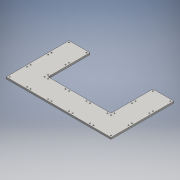
# Autodesk Inventor part: InnerFrame
Saved by Autodesk Inventor 2016 (Build 200138000, 138)
## iProperties
Created: 2016-05-22
Part Number: InnerFrame
Material: Generic
Document SubType Name: Modeling
Designer: Kurtis
Density: 1 g/cm^3
Appearance: Default
Author: Kurtis
Autodesk Inventor part; units mm, degrees
ref_plane "YZ Plane" through (0, 0, 0) normal (1, 0, 0) x (0, 1, 0)
ref_plane "XZ Plane" through (0, 0, 0) normal (0, 1, 0) x (-1, 0, 0)
ref_plane "XY Plane" through (0, 0, 0) normal (0, 0, 1) x (1, 0, 0)
sketch "Sketch1" plane through (0, 0, 0) normal (0, 0, 1) x (1, 0, 0)
  line L0 (0, 0) -> (0, 180)
  line L1 (0, 180) -> (60, 180)
  line L2 (60, 180) -> (60, 60)
  line L3 (60, 60) -> (240, 60)
  line L4 (240, 60) -> (240, 180)
  line L5 (240, 180) -> (300, 180)
  line L6 (300, 180) -> (300, 0)
  line L7 (300, 0) -> (0, 0)
  line L8 (60, 60) -> (0, 60) construction
  line L9 (60, 60) -> (60, 0) construction
  line L10 (240, 60) -> (300, 60) construction
  line L11 (240, 60) -> (240, 0) construction
  line L12 (240, 60) -> (180, 60) construction
  line L13 (180, 60) -> (180, 0) construction
  line L14 (180, 60) -> (120, 60) construction
  line L15 (120, 60) -> (120, 0) construction
  line L16 (240, 60) -> (240, 120) construction
  line L17 (240, 120) -> (300, 120) construction
  line L18 (60, 60) -> (60, 120) construction
  line L19 (60, 120) -> (0, 120) construction
  line L20 (0, 120) -> (60, 180) construction
  line L21 (0, 60) -> (60, 120) construction
  line L22 (0, 0) -> (60, 60) construction
  line L23 (60, 0) -> (120, 60) construction
  line L24 (120, 0) -> (180, 60) construction
  line L25 (180, 0) -> (240, 60) construction
  line L26 (240, 0) -> (300, 60) construction
  line L27 (240, 60) -> (300, 120) construction
  line L28 (240, 120) -> (300, 180) construction
  line L29 (5, 175) -> (55, 175) construction
  line L30 (55, 175) -> (55, 125) construction
  line L31 (55, 125) -> (5, 125) construction
  line L32 (5, 125) -> (5, 175) construction
  line L33 (5, 175) -> (55, 125) construction
  line L34 (55, 175) -> (5, 125) construction
  line L35 (5, 115) -> (55, 115) construction
  line L36 (55, 115) -> (55, 65) construction
  line L37 (55, 65) -> (5, 65) construction
  line L38 (5, 65) -> (5, 115) construction
  line L39 (5, 115) -> (55, 65) construction
  line L40 (55, 115) -> (5, 65) construction
  line L41 (5, 55) -> (55, 55) construction
  line L42 (55, 55) -> (55, 5) construction
  line L43 (55, 5) -> (5, 5) construction
  line L44 (5, 5) -> (5, 55) construction
  line L45 (5, 55) -> (55, 5) construction
  line L46 (55, 55) -> (5, 5) construction
  line L47 (65, 55) -> (115, 55) construction
  line L48 (115, 55) -> (115, 5) construction
  line L49 (115, 5) -> (65, 5) construction
  line L50 (65, 5) -> (65, 55) construction
  line L51 (65, 55) -> (115, 5) construction
  line L52 (115, 55) -> (65, 5) construction
  line L53 (125, 5) -> (175, 5) construction
  line L54 (175, 5) -> (175, 55) construction
  line L55 (175, 55) -> (125, 55) construction
  line L56 (125, 55) -> (125, 5) construction
  line L57 (125, 5) -> (175, 55) construction
  line L58 (175, 5) -> (125, 55) construction
  line L59 (185, 5) -> (235, 5) construction
  line L60 (235, 5) -> (235, 55) construction
  line L61 (235, 55) -> (185, 55) construction
  line L62 (185, 55) -> (185, 5) construction
  line L63 (185, 5) -> (235, 55) construction
  line L64 (235, 5) -> (185, 55) construction
  line L65 (245, 5) -> (295, 5) construction
  line L66 (295, 5) -> (295, 55) construction
  line L67 (295, 55) -> (245, 55) construction
  line L68 (245, 55) -> (245, 5) construction
  line L69 (245, 5) -> (295, 55) construction
  line L70 (295, 5) -> (245, 55) construction
  line L71 (295, 65) -> (245, 65) construction
  line L72 (245, 65) -> (245, 115) construction
  line L73 (245, 115) -> (295, 115) construction
  line L74 (295, 115) -> (295, 65) construction
  line L75 (295, 65) -> (245, 115) construction
  line L76 (245, 65) -> (295, 115) construction
  line L77 (245, 125) -> (295, 125) construction
  line L78 (295, 125) -> (295, 175) construction
  line L79 (295, 175) -> (245, 175) construction
  line L80 (245, 175) -> (245, 125) construction
  line L81 (245, 125) -> (295, 175) construction
  line L82 (295, 125) -> (245, 175) construction
  circle A0 centre (245, 175) radius 1.5
  circle A1 centre (295, 175) radius 1.5
  circle A2 centre (295, 125) radius 1.5
  circle A3 centre (245, 125) radius 1.5
  circle A4 centre (245, 115) radius 1.5
  circle A5 centre (295, 115) radius 1.5
  circle A6 centre (295, 65) radius 1.5
  circle A7 centre (245, 65) radius 1.5
  circle A8 centre (245, 55) radius 1.5
  circle A9 centre (295, 55) radius 1.5
  circle A10 centre (295, 5) radius 1.5
  circle A11 centre (245, 5) radius 1.5
  circle A12 centre (235, 55) radius 1.5
  circle A13 centre (185, 55) radius 1.5
  circle A14 centre (185, 5) radius 1.5
  circle A15 centre (235, 5) radius 1.5
  circle A16 centre (125, 55) radius 1.5
  circle A17 centre (175, 55) radius 1.5
  circle A18 centre (175, 5) radius 1.5
  circle A19 centre (125, 5) radius 1.5
  circle A20 centre (115, 55) radius 1.5
  circle A21 centre (65, 55) radius 1.5
  circle A22 centre (65, 5) radius 1.5
  circle A23 centre (115, 5) radius 1.5
  circle A24 centre (5, 55) radius 1.5
  circle A25 centre (55, 55) radius 1.5
  circle A26 centre (55, 5) radius 1.5
  circle A27 centre (5, 5) radius 1.5
  circle A28 centre (5, 65) radius 1.5
  circle A29 centre (55, 65) radius 1.5
  circle A30 centre (5, 115) radius 1.5
  circle A31 centre (55, 115) radius 1.5
  circle A32 centre (5, 125) radius 1.5
  circle A33 centre (55, 125) radius 1.5
  circle A34 centre (5, 175) radius 1.5
  circle A35 centre (55, 175) radius 1.5
  point P0 (30, 150)
  point P1 (30, 90)
  point P2 (30, 30)
  point P3 (90, 30)
  point P4 (150, 30)
  point P5 (210, 30)
  point P6 (270, 30)
  point P7 (270, 90)
  point P8 (270, 150)
  dimension "d0" = 180
  dimension "d1" = 60
  dimension "d2" = 120
  dimension "d3" = 180
  dimension "d4" = 60
  dimension "d5" = 60
  dimension "d6" = 60
  dimension "d7" = 60
  dimension "d8" = 60
  dimension "d9" = 50
  dimension "d10" = 50
  dimension "d11" = 50
  dimension "d12" = 50
  dimension "d13" = 50
  dimension "d14" = 50
  dimension "d15" = 50
  dimension "d16" = 50
  dimension "d17" = 50
  dimension "d18" = 50
  dimension "d19" = 50
  dimension "d20" = 50
  dimension "d21" = 50
  dimension "d22" = 50
  dimension "d23" = 50
  dimension "d24" = 50
  dimension "d25" = 50
  dimension "d26" = 50
  dimension "d27" = 3
  dimension "d28" = 3
  dimension "d29" = 3
  dimension "d30" = 3
  dimension "d31" = 3
  dimension "d32" = 3
  dimension "d33" = 3
  dimension "d34" = 3
  dimension "d35" = 3
  dimension "d36" = 3
  dimension "d37" = 3
  dimension "d38" = 3
  dimension "d39" = 3
  dimension "d40" = 3
  dimension "d41" = 3
  dimension "d42" = 3
  dimension "d43" = 3
  dimension "d44" = 3
  dimension "d45" = 3
  dimension "d46" = 3
  dimension "d47" = 3
  dimension "d48" = 3
  dimension "d49" = 3
  dimension "d50" = 3
  dimension "d51" = 3
  dimension "d52" = 3
  dimension "d53" = 3
  dimension "d54" = 3
  dimension "d55" = 3
  dimension "d56" = 3
  dimension "d57" = 3
  dimension "d58" = 3
  dimension "d59" = 3
  dimension "d60" = 3
  dimension "d61" = 3
  dimension "d62" = 3
  constraints: 166 end point, 36 centre point, 36 coincident, 29 midpoint, 18 parallel, 18 perpendicular, 17 point on line, 9 horizontal, 1 vertical
  measures "d0" distance of L0.start L0.end
  measures "d1" distance of L0.end L1.end
  measures "d2" distance of L1.end L2.end
  measures "d3" distance of L2.end L3.end
  measures "d4" distance of L4.end L5.end
  measures "d5" distance of L3.end L12.end
  measures "d6" distance of L12.end L14.end
  measures "d7" distance of L3.end L16.end
  measures "d8" distance of L2.end L18.end
  measures "d9" distance of L30.end L31.end
  measures "d10" distance of L29.end L30.end
  measures "d11" distance of L36.end L37.end
  measures "d12" distance of L35.end L36.end
  measures "d13" distance of L42.end L43.end
  measures "d14" distance of L41.end L42.end
  measures "d15" distance of L48.end L49.end
  measures "d16" distance of L47.end L48.end
  measures "d17" distance of L55.end L54.end
  measures "d18" distance of L54.end L53.end
  measures "d19" distance of L61.end L60.end
  measures "d20" distance of L60.end L59.end
  measures "d21" distance of L67.end L66.end
  measures "d22" distance of L66.end L65.end
  measures "d23" distance of L72.end L73.end
  measures "d24" distance of L71.end L72.end
  measures "d25" distance of L79.end L78.end
  measures "d26" distance of L78.end L77.end
  measures "d27" diameter of A0
  measures "d28" diameter of A1
  measures "d29" diameter of A2
  measures "d30" diameter of A3
  measures "d31" diameter of A4
  measures "d32" diameter of A5
  measures "d33" diameter of A6
  measures "d34" diameter of A7
  measures "d35" diameter of A8
  measures "d36" diameter of A9
  measures "d37" diameter of A10
  measures "d38" diameter of A11
  measures "d39" diameter of A12
  measures "d40" diameter of A13
  measures "d41" diameter of A14
  measures "d42" diameter of A15
  measures "d43" diameter of A16
  measures "d44" diameter of A17
  measures "d45" diameter of A18
  measures "d46" diameter of A19
  measures "d47" diameter of A20
  measures "d48" diameter of A21
  measures "d49" diameter of A22
  measures "d50" diameter of A23
  measures "d51" diameter of A24
  measures "d52" diameter of A25
  measures "d53" diameter of A26
  measures "d54" diameter of A27
  measures "d55" diameter of A28
  measures "d56" diameter of A29
  measures "d57" diameter of A30
  measures "d58" diameter of A31
  measures "d59" diameter of A32
  measures "d60" diameter of A33
  measures "d61" diameter of A34
  measures "d62" diameter of A35
extrude "Extrusion1" add sketch "Sketch1" along normal blind 5
body "Solid1"
